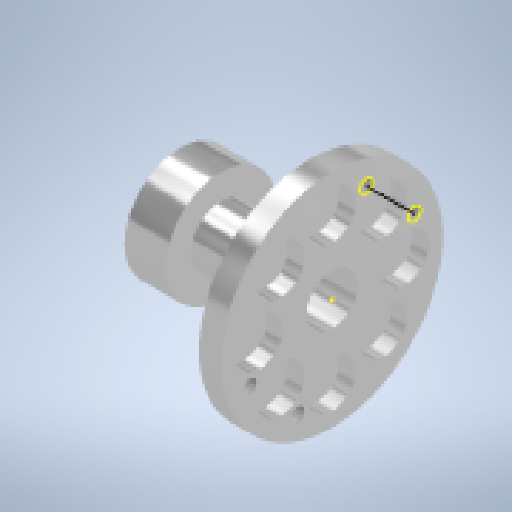
# Autodesk Inventor part: P411
Saved by Autodesk Inventor 2023 (Build 270158000, 158)
## iProperties
Created: 2022-09-14
Part Number: P411
Material: Aluminum 6061
Document SubType Name: Modeling
Designer: D.C. Eksteen
Density: 2.7 g/cm^3
Appearance: Aluminum - Flat
Author: D.C. Eksteen
Title: BEARING AND DISC
Autodesk Inventor part; units mm, degrees
ref_plane "YZ Plane" through (0, 0, 0) normal (1, 0, 0) x (0, 1, 0)
ref_plane "XZ Plane" through (0, 0, 0) normal (0, 1, 0) x (-1, 0, 0)
sketch "Sketch1" plane through (0, 0, 0) normal (1, 0, 0) x (0, 1, 0)
  circle A0 centre (0, 0) radius 35
  circle A1 centre (0, 0) radius 8
  dimension "d0" = 70
  dimension "d1" = 16
  constraints: 2 centre point, 2 coincident
  measures "d0" diameter of A0
  measures "d1" diameter of A1
extrude "Extrusion1" add sketch "Sketch1" along normal blind 7
sketch "Sketch2" plane through (7, 0, 0) normal (1, 0, 0) x (0, 0, -1)
  circle A0 centre (0, 0) radius 23 construction
  point P0 (-23, 0)
  point P1 (-16.2635, -16.2635)
  point P2 (0, -23)
  point P3 (16.2635, -16.2635)
  point P4 (23, 0)
  point P5 (16.2635, 16.2635)
  point P6 (0, 23)
  point P7 (-16.2635, 16.2635)
  dimension "d4" = 46
  dimension "d5" = 0
  dimension "d8" = 360
  constraints: 1 coincident, 1 horizontal alignment, 11 other
  measures "d5" vertical distance of point (0, 0) point (-23, 0)
hole "Hole1" at (7, 0, 23) at (7, -16.2635, 16.2635) at (7, -23, 0) at (7, -16.2635, -16.2635) at (7, 0, -23) at (7, 16.2635, -16.2635) at (7, 23, 0) at (7, 16.2635, 16.2635) direction (-1, 0, 0) diameter 15 depth 5
sketch "Sketch3" plane through (0, 0, 0) normal (-1, 0, 0) x (0, 0, 1)
  circle A0 centre (0, 0) radius 35 projected
  circle A1 centre (0, 0) radius 8 projected
  circle A2 centre (0, 0) radius 9.5
  dimension "d17" = 19
  constraints: 1 centre point, 1 coincident
  measures "d17" diameter of A2
extrude "Extrusion2" add sketch "Sketch3" along normal blind 28 contours A2
sketch "Sketch4" plane through (0, 0, 0) normal (-1, 0, 0) x (0, 0, 1)
  circle A0 centre (0, 0) radius 11
  circle A1 centre (0, 0) radius 9.5 projected
  dimension "d20" = 22
  constraints: 1 centre point, 1 coincident
  measures "d20" diameter of A0
extrude "Extrusion3" add sketch "Sketch4" along normal blind 3
sketch "Sketch5" plane through (-28, 0, 0) normal (-1, 0, 0) x (0, 0, 1)
  circle A0 centre (0, 0) radius 17.5
  circle A1 centre (0, 0) radius 8 projected
  dimension "d23" = 35
  constraints: 1 centre point, 1 coincident
  measures "d23" diameter of A0
extrude "Extrusion4" add sketch "Sketch5" along normal blind 2
sketch "Sketch6" plane through (-30, 0, 0) normal (-1, 0, 0) x (0, 0, 1)
  circle A0 centre (0, 0) radius 17.5
  circle A1 centre (0, 0) radius 8 projected
  circle A2 centre (0, 0) radius 14
  dimension "d26" = 28
  dimension "d27" = 35
  constraints: 2 centre point, 2 coincident
  measures "d26" diameter of A2
  measures "d27" diameter of A0
extrude "Extrusion5" add sketch "Sketch6" along normal blind 11 contours A0
ref_plane "Work Plane1" through (-38.5, 0, 0) normal (-1, 0, 0) x (0, 0, 1)
sketch "Sketch7" plane through (-38.5, 0, 0) normal (-1, 0, 0) x (0, 0, 1)
  circle A0 centre (0, 0) radius 14 projected
  circle A1 centre (0, 0) radius 14.7
  dimension "d31" = 29.4
  constraints: 1 centre point, 1 coincident
  measures "d31" diameter of A1
extrude "Extrusion6" cut sketch "Sketch7" against normal blind 1.3
sketch "Sketch12" plane through (7, 0, 0) normal (1, 0, 0) x (0, 0, -1)
  circle A0 centre (0, 23) radius 7.5 projected
  circle A1 centre (23, 0) radius 7.5 projected
  circle A2 centre (0, -23) radius 7.5 projected
  circle A3 centre (-23, 0) radius 7.5 projected
  circle A4 centre (-16.2635, -16.2635) radius 7.5 projected
  circle A5 centre (16.2635, -16.2635) radius 7.5 projected
  circle A6 centre (16.2635, 16.2635) radius 7.5 projected
  circle A7 centre (-16.2635, 16.2635) radius 7.5 projected
  circle A8 centre (0, 0) radius 35 projected
  circle A9 centre (0, 0) radius 8 projected
  circle A10 centre (0, 0) radius 28 construction
  line L0 (-16.2635, 16.2635) -> (16.2635, -16.2635) construction
  line L1 (0, 0) -> (0, 23)
  line L2 (0, 0) -> (10.7151, 25.8686)
  line L3 (0, 0) -> (25.8686, 10.7151)
  point P0 (-25.8686, -10.7151)
  point P1 (-10.7151, -25.8686)
  dimension "d41" = 56
  dimension "d42" = 22.5
  dimension "d43" = 45
  constraints: 8 end point, 3 coincident, 2 point on circle, 2 symmetric about line, 1 centre point, 1 vertical
  measures "d41" diameter of A10
  measures "d42" angle of L1 L2
  measures "d43" angle of L2 L3
hole "Hole3" at (7, 25.8686, -10.7151) at (7, 10.7151, -25.8686) at (7, -25.8686, 10.7151) at (7, -10.7151, 25.8686) direction (-1, 0, 0) diameter 4.134 depth 14.2 tip angle 118 thread size "M5x0.8" class "6H" standard "ANSI Metric M Profile"
sketch "Sketch13" plane through (7, 0, 0) normal (1, 0, 0) x (0, 0, -1)
  circle A0 centre (10.7151, 25.8686) radius 2.067 projected
  circle A1 centre (25.8686, 10.7151) radius 2.067 projected
  line L0 (10.7151, 25.8686) -> (25.8686, 10.7151)
  point P0 (0, 0)
  constraints: 2 end point
body "Solid1"
